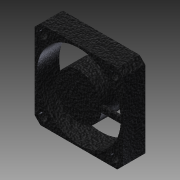
# Autodesk Inventor part: Fan
Saved by Autodesk Inventor 2013 (Build 170138000, 138)
## iProperties
Created: 2014-11-16
Part Number: Fan
Material: Generic
Document SubType Name: Modeling
Designer: Kyle
Density: 1 g/cm^3
Author: Kyle
Autodesk Inventor part; units mm, degrees
ref_plane "YZ Plane" through (0, 0, 0) normal (1, 0, 0) x (0, 1, 0)
ref_plane "XZ Plane" through (0, 0, 0) normal (0, 1, 0) x (-1, 0, 0)
ref_plane "XY Plane" through (0, 0, 0) normal (0, 0, 1) x (1, 0, 0)
sketch "Sketch1" plane through (0, 0, 0) normal (0, 0, 1) x (1, 0, 0)
  line L0 (0, 0) -> (40.005, 0)
  line L1 (40.005, 0) -> (40.005, -40.005)
  line L2 (40.005, -40.005) -> (0, -40.005)
  line L3 (0, -40.005) -> (0, 0)
  dimension "d0" = 40.005
  dimension "d1" = 40.005
  constraints: 8 end point, 2 parallel, 1 horizontal, 1 perpendicular
  measures "d0" distance of L2.end L0.start
  measures "d1" distance of L0.start L0.end
extrude "Extrusion1" add sketch "Sketch1" along normal blind 10.16
sketch "Sketch2" plane through (0, 0, 10.16) normal (0, 0, 1) x (1, 0, 0)
  line L0 (40.005, 0) -> (0, 0) projected
  line L1 (0, 0) -> (0, -40.005) projected
  line L2 (0, -40.005) -> (40.005, -40.005) projected
  line L3 (40.005, -40.005) -> (40.005, 0) projected
  circle A0 centre (20.0025, -20.0025) radius 19.05
  circle A1 centre (3.81, -3.81) radius 1.778
  circle A2 centre (36.195, -3.81) radius 1.778
  circle A3 centre (36.195, -36.195) radius 1.778
  circle A4 centre (3.81, -36.195) radius 1.778
  dimension "d4" = 38.1
  dimension "d6" = 3.81
  dimension "d7" = 3.81
  dimension "d8" = 3.81
  dimension "d9" = 3.81
  dimension "d10" = 3.556
  dimension "d11" = 3.556
  dimension "d12" = 3.556
  dimension "d13" = 3.556
  constraints: 5 centre point, 4 coincident
  measures "d4" diameter of A0
  measures "d6" distance from line of L2 point (3.81, -36.195)
  measures "d7" distance from line of L1 point (3.81, -36.195)
  measures "d8" distance from line of L3 point (36.195, -3.81)
  measures "d9" distance from line of L0 point (36.195, -3.81)
  measures "d10" diameter of A4
  measures "d11" diameter of A1
  measures "d12" diameter of A2
  measures "d13" diameter of A3
extrude "Extrusion2" cut sketch "Sketch2" against normal blind 12.7 contours A0 | A1 | A2 | A3 | A4
sketch "Sketch3" plane through (0, 0, 10.16) normal (0, 0, 1) x (1, 0, 0)
  circle A0 centre (20.0025, -20.0025) radius 19.05 projected
  circle A1 centre (20.0025, -20.0025) radius 10.287
  dimension "d16" = 20.574
  constraints: 1 centre point, 1 coincident
  measures "d16" diameter of A1
extrude "Extrusion3" add sketch "Sketch3" against normal blind 10.16 contours A1
sketch "Sketch4" plane through (40.005, -40.005, 0) normal (1, 0, 0) x (0, 0, -1)
  line L0 (-10.16, 0) -> (-10.16, 40.005) projected
  line L1 (-10.16, 21.2725) -> (-8.89, 21.2725)
  line L2 (-8.89, 21.2725) -> (-8.89, 18.7325)
  line L3 (-8.89, 18.7325) -> (-10.16, 18.7325)
  line L4 (-10.16, 18.7325) -> (-10.16, 21.2725)
  point P0 (-10.16, 20.0025)
  dimension "d20" = 1.27
  dimension "d21" = 1.27
  dimension "d22" = 1.27
  constraints: 8 end point, 2 parallel, 2 point on line, 1 horizontal, 1 midpoint, 1 perpendicular
  measures "d20" distance of L1.start point (-10.16, 20.002)
  measures "d21" distance of point (-10.16, 18.732) point (-10.16, 20.002)
  measures "d22" distance of L1.start L1.end
extrude "Extrusion4" add sketch "Sketch4" against normal blind 10.16
chamfer "Chamfer1" distance 2.54 angle 45 4 edges at (0, 0, 5.08) (40.005, 0, 5.08) (40.005, -40.005, 5.08) (0, -40.005, 5.08)
body "Solid1"
